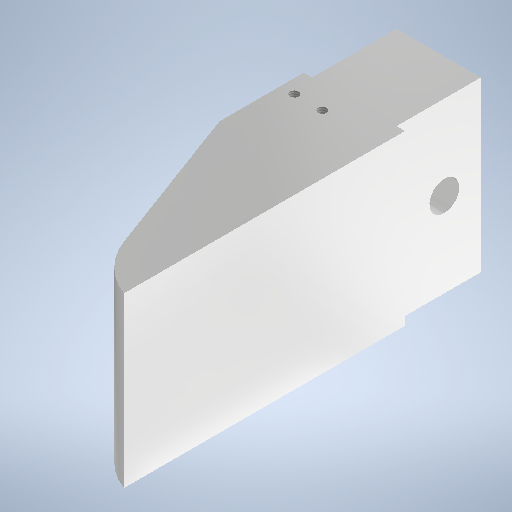
# Autodesk Inventor part: MontageAufnahmeLO
Saved by Autodesk Inventor 2025 (Build 290162010, 162A)
## iProperties
Created: 2024-11-18
Part Number: MontageAufnahmeLO
Material: PC/ABS-Kunststoff, 3DDruck, PLA
Document SubType Name: Modeling
Designer: Admin
Density: 1.1 g/cm^3
Appearance: Glatt - Weiß(2)
Mass: 29.2248 g
Surface Area: 64.7654 cm^2
Volume: 26.568 cm^3
Author: Admin
Autodesk Inventor part; units mm, degrees
ref_plane "YZ Plane" through (0, 0, 0) normal (1, 0, 0) x (0, 1, 0)
ref_plane "XZ Plane" through (0, 0, 0) normal (0, 1, 0) x (-1, 0, 0)
ref_plane "XY Plane" through (0, 0, 0) normal (0, 0, 1) x (1, 0, 0)
sketch "Skizze1" plane through (0, 0, 0) normal (0, 0, 1) x (1, 0, 0)
  line L0 (-9, 0) -> (9, 0) construction
  arc A0 (1.0455, -58.0455) -> (9, -66) centre (13.7004, -53.345) ccw
  line L1 (1.0455, -58.0455) -> (9, -58.0455) construction
  line L2 (9, -66) -> (9, -58.0455)
  line L3 (9, -66) -> (4, -66) construction
  line L4 (9, -16) -> (9, -58.0455)
  line L5 (-9, -31) -> (1.0455, -58.0455)
  line L6 (7.5, 1) -> (-7.5, 1) projected
  line L7 (-7.5, 1) -> (-7.5, 16) projected
  line L8 (-7.5, 16) -> (-9, 16) projected
  line L9 (-9, 16) -> (-9, -16) projected
  line L10 (-9, -16) -> (-7.5, -16) projected
  line L11 (-7.5, -16) -> (-7.5, -1) projected
  line L12 (-7.5, -1) -> (7.5, -1) projected
  line L13 (7.5, -1) -> (7.5, -16) projected
  line L14 (7.5, -16) -> (9, -16) projected
  line L15 (9, -16) -> (9, 16) projected
  line L16 (9, 16) -> (7.5, 16) projected
  line L17 (7.5, 16) -> (7.5, 1) projected
  line L18 (-9, -16) -> (-9, -31)
  point P0 (0, 0)
  dimension "d0" = 5
  dimension "d1" = 50
  dimension "d4" = 15
  constraints: 14 end point, 2 midpoint, 2 perpendicular, 2 point on circle, 2 vertical, 1 centre point, 1 coincident, 1 collinear, 1 horizontal, 1 point on line, 1 tangent
  measures "d0" distance of L3.start L3.end
  measures "d1" distance of L4.start L3.start
  measures "d4" distance of L9.end L5.start
extrude "Extrusion1" add sketch "Skizze1" against normal blind 30 contours L5 L18 L10 L11 L12 L13 L14 L4 L2 A0
sketch "Skizze3" plane through (0, 0, 0) normal (0, 0, 1) x (1, 0, 0)
  circle A0 centre (-13.05, -20.1503) radius 1.621 construction
  line L0 (-13.05, -20.1503) -> (-6.55, -20.1503) construction
  line L1 (-6.55, -20.1503) -> (-1.55, -20.1503) construction
  point P0 (0, 0)
  dimension "d1" = 50
  dimension "d14" = 6.5
  dimension "d15" = 5
  constraints: 4 coincident, 4 end point, 1 horizontal, 1 point on line
  measures "d14" distance of L0.start L0.end
  measures "d15" distance of L0.end L1.end
hole "Bohrung2" at (-6.55, -20.1503, 0) at (-1.55, -20.1503, 0) direction (0, 0, -1) diameter 1.567 depth 10 tip angle 118 thread size "M2x0.4" class "6H" standard "ANSI Metric M Profile"
sketch "Skizze4" plane through (-7.5, -16, 0) normal (-1, 0, 0) x (0, 0, 1)
  circle A0 centre (-15, 8.5) radius 2.5 projected
  point P0 (0, 16)
hole "Bohrung3" at (-7.5, -7.5, -15) direction (1, 0, 0) diameter 5.3 end through all clearance for "Flachkopfmaschinenschraube" size "M5" standard "ANSI Metrisches M Profil"
